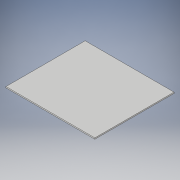
# Autodesk Inventor part: top
Saved by Autodesk Inventor 2017 (Build 210142000, 142)
## iProperties
Created: 2017-03-16
Part Number: top
Material: Generic
Document SubType Name: Modeling
Designer: LaFaucheuse
Density: 1 g/cm^3
Appearance: Default
Author: LaFaucheuse
Autodesk Inventor part; units mm, degrees
ref_plane "YZ Plane" through (0, 0, 0) normal (1, 0, 0) x (0, 1, 0)
ref_plane "XZ Plane" through (0, 0, 0) normal (0, 1, 0) x (-1, 0, 0)
ref_plane "XY Plane" through (0, 0, 0) normal (0, 0, 1) x (1, 0, 0)
sketch "Esquisse1" plane through (0, 0, 0) normal (0, 1, 0) x (-1, 0, 0)
  line L0 (0, 0) -> (224.368, 0)
  line L1 (224.368, 0) -> (224.368, -200)
  line L2 (224.368, -200) -> (0, -200)
  line L3 (0, -200) -> (0, 0)
  dimension "d0" = 224.368
  dimension "d1" = 200
  constraints: 8 end point, 2 parallel, 1 horizontal, 1 perpendicular
  measures "d0" distance of L0.start L0.end
  measures "d1" distance of L2.end L0.start
extrude "Extrusion1" add sketch "Esquisse1" along normal blind 3
